# Autodesk Inventor part: Zahnriemen
Saved by Autodesk Inventor 2016 (Build 200138000, 138)
## iProperties
Created: 2015-08-24
Part Number: Zahnriemen
Material: Rubber
Document SubType Name: Modeling
Designer: 4ndreas
Density: 1 g/cm^3
Appearance: Rubber - Black - Version 1.1
CustomPartVersion: 1
Author: 4ndreas
Autodesk Inventor part; units mm, degrees
sketch "Skizzenpfad" plane through (0, 0, 0) normal (0, 0, 1) x (1, 0, 0)
  arc A0 (-62.2966, 30.7178) -> (-61.9196, -30.4355) centre (-85, 0) ccw
  arc A1 (-27.7306, 5.1701) -> (-20.6178, 4.4524) centre (-23.57, 10.7995) ccw
  arc A2 (-5.7791, -11.3453) -> (-5.3697, 11.5447) centre (0, 0) ccw
  arc A3 (-20.3927, -3.9013) -> (-27.7997, -4.5611) centre (-23.57, -10.1387) ccw
  line L0 (-27.7997, -4.5611) -> (-61.9196, -30.4355)
  line L1 (-62.2966, 30.7178) -> (-27.7306, 5.1701)
  line L2 (-20.6178, 4.4524) -> (-5.3697, 11.5447)
  line L3 (-5.7791, -11.3453) -> (-20.3927, -3.9013)
  constraints: 8 end point, 8 point on circle, 4 centre point
ref_plane "Querschnittsebene" through (-61.9196, -30.4355, 0) normal (0.7968, 0.6042, 0) x (0, 0, 1)
ref_plane "Arbeitsebene2" through (-85, 0, 0) normal (-1, 0, 0) x (0, 0, 1)
ref_plane "Arbeitsebene3" through (0, 0, 0) normal (-0.9857, -0.1686, 0) x (0, 0, 1)
sketch "Querschnitt" plane through (-61.9196, -30.4355, 0) normal (0.7968, 0.6042, 0) x (0, 0, 1)
  line L0 (-5, 0.5) -> (5, 0.5)
  line L1 (5, 0.5) -> (5, -0.5)
  line L2 (5, -0.5) -> (-5, -0.5)
  line L3 (-5, -0.5) -> (-5, 0.5)
  line L4 (-5, 0) -> (5, 0) construction
  point P0 (0, 0)
  point P1 (0, 0)
  dimension "d0" = 10
  dimension "d4" = 0.5
  dimension "d5" = 0.5
  constraints: 10 end point, 3 midpoint, 2 parallel, 1 coincident, 1 horizontal, 1 perpendicular, 1 other
  measures "d0" distance between parallel lines of L1 L3
  measures "d4" distance between parallel lines of L2 L4
  measures "d5" distance between parallel lines of L4 L0
sweep "Riemen" add profiles "Querschnitt" path "Skizzenpfad"
equation "\"d0\" = da_B"
equation "\"d4\" = da_a"
equation "\"d5\" = da_a2"
equation "\"da_B\" = 10"
equation "\"da_pb\" = 5"
equation "\"da_L\" = 355"
equation "\"da_a\" = 0.5"
equation "\"da_S\" = 2.65"
equation "\"da_Beta\" = 20deg"
equation "\"da_Ht\" = 1.2"
equation "\"da_H\" = 2.2"
equation "\"da_a2\" = 0.5"
body "Solid1"
